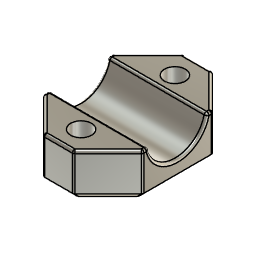
GPS_CLAMP_LOW (Autodesk Fusion 360 design; units mm, degrees)
Autodesk Fusion 360 part; units mm, degrees
note: some values were not read from the file. Set by a fixed rule: which sketch regions a step uses.
sketch "Esquisse1" plane through (0, 0, 0) normal (0, 0, 1) x (1, 0, 0)
  line L0 (7, 0) -> (13, 0)
  line L1 (20, 7) -> (20, 21)
  line L2 (13, 28) -> (7, 28)
  line L3 (0, 21) -> (0, 7)
  line L4 (10, 28) -> (10, 0) construction
  circle A0 centre (10, 23.45) radius 2.1
  circle A1 centre (10, 4.55) radius 2.1
  line L5 (-6, 20) -> (25, 20) construction
  line L6 (25, 20) -> (25, 8) construction
  line L7 (25, 8) -> (-6, 8) construction
  line L8 (-6, 8) -> (-6, 20) construction
  line L9 (13, 0) -> (20, 7)
  line L10 (7, 0) -> (0, 7)
  line L11 (20, 21) -> (13, 28)
  line L12 (7, 28) -> (0, 21)
  point P0 (20, 0)
  point P1 (20, 28)
  point P2 (0, 28)
  dimension "d1" = 20
  dimension "d2" = 28
  dimension "d3" = 4.2
  dimension "d4" = 4.2
  dimension "d5" = 18.9
  dimension "d6" = 4.55
  dimension "d7" = 12
  dimension "d8" = 8
  dimension "d9" = 7
  dimension "d10" = 7
  dimension "d11" = 7
  dimension "d12" = 7
  dimension "d13" = 7
  dimension "d14" = 7
  dimension "d15" = 7
  dimension "d16" = 7
  constraint horizontal L0
  constraint vertical L1
  constraint horizontal L2
  constraint vertical L3
  constraint coincident L4 A0.centre
  constraint coincident L4 A1.centre
  constraint horizontal L5
  constraint vertical L6
  constraint horizontal L7
  constraint vertical L8
  constraint coincident L0 L4.end
  constraint coincident P0 L0
  constraint coincident P0 L1
  constraint coincident origin L0
  constraint coincident origin L3
  constraint coincident L2 L4.start
  constraint coincident P1 L1
  constraint coincident P1 L2
  constraint coincident P2 L2
  constraint coincident P2 L3
  measures "d1" distance of origin P0
  measures "d2" distance of origin P2
  measures "d3" diameter of A0
  measures "d4" diameter of A1
  measures "d5" distance of A0.centre A1.centre
  measures "d6" distance of L0 A1.centre
  measures "d7" distance of L5.start L7.end
  measures "d8" distance of origin L7
  measures "d9" distance of P0 L0.end
  measures "d10" distance of P0 L1.start
  measures "d11" distance of origin L0.start
  measures "d12" distance of origin L3.end
  measures "d13" distance of P1 L1.end
  measures "d14" distance of P1 L2.start
  measures "d15" distance of P2 L2.end
  measures "d16" distance of P2 L3.start
extrude "Extrusion1" add sketch "Esquisse1" along normal blind 9
sketch "Esquisse2" plane through (20, 0, 0) normal (1, 0, 0) x (0, 1, 0)
  line L0 (7, 0) -> (21, 0)
  line L1 (21, 0) -> (21, 9)
  line L2 (21, 9) -> (7, 9)
  line L3 (7, 9) -> (7, 0)
  circle A0 centre (14, 10) radius 6
  dimension "d19" = 12
  dimension "d20" = 10
  dimension "d21" = 7
  measures "d19" diameter of A0
  measures "d20" distance of L0 A0.centre
  measures "d21" distance of L3 A0.centre
extrude "Extrusion2" cut sketch "Esquisse2" against normal blind 20 contours L2 A0 | L2 A0
chamfer "Chanfrein1" distance 1.5 angle 45 8 edges at (16.5, 3.5, 0) (20, 14, 0) (16.5, 24.5, 0) (10, 28, 0) (3.5, 24.5, 0) (0, 14, 0) (3.5, 3.5, 0) (10, 0, 0)
fillet "Congé1" radius 0.5 22 edges at (10, 8.0839, 9) (10, 19.9161, 9) (0, 21, 5.25) (0, 7, 5.25) (0, 7.542, 9) (7, 0, 5.25) (13, 0, 5.25) (20, 7, 5.25) (20, 7.542, 9) (20, 14, 4) (0, 14, 4) (3.5, 24.5, 9) (10, 28, 9) (16.5, 24.5, 9) (20, 20.458, 9) (0, 20.458, 9) (20, 21, 5.25) (13, 28, 5.25) (7, 28, 5.25) (16.5, 3.5, 9) (10, 0, 9) (3.5, 3.5, 9)
fillet "Congé2" radius 0.5 8 edges at (0.769, 7.3185, 0.731) (7.3185, 0.769, 0.731) (12.6815, 0.769, 0.731) (0.769, 20.6815, 0.731) (7.3185, 27.231, 0.731) (12.6815, 27.231, 0.731) (19.231, 20.6815, 0.731) (19.231, 7.3185, 0.731)
equation "d5 = 14.7 mm + 4.2 mm"
equation "d6 = ( ( 28 - 18.9 ) / 2 ) * 1 mm"
equation "d10 = d9"
equation "d12 = d11"
equation "d14 = d13"
equation "d16 = d15"
